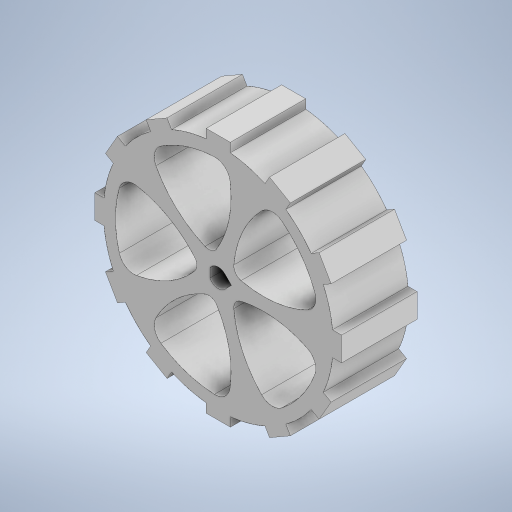
# Autodesk Inventor part: Drive_Wheel
Saved by Autodesk Inventor 2024 (Build 280153000, 153)
## iProperties
Created: 2024-04-15
Part Number: Drive_Wheel
Material: Generic
Document SubType Name: Modeling
Designer: CJ110
Density: 1 g/cm^3
Appearance: Default
Author: CJ110
Autodesk Inventor part; units mm, degrees
ref_plane "YZ Plane" through (0, 0, 0) normal (1, 0, 0) x (0, 1, 0)
ref_plane "XZ Plane" through (0, 0, 0) normal (0, 1, 0) x (-1, 0, 0)
ref_plane "XY Plane" through (0, 0, 0) normal (0, 0, 1) x (1, 0, 0)
sketch "Sketch1" plane through (0, 0, 0) normal (0, 0, 1) x (1, 0, 0)
  circle A0 centre (0, 0) radius 38.1
  circle A1 centre (0, 0) radius 3.1
  line L0 (-2.75, 1.4309) -> (-2.75, -1.4309)
  line L1 (2.192, 2.192) -> (4.3841, 0)
  line L2 (4.3841, 0) -> (2.192, -2.192)
  dimension "d0" = 76.2
  dimension "d1" = 6.2
  dimension "d2" = 2.75
  constraints: 6 end point, 4 point on circle, 2 centre point, 2 coincident, 2 tangent, 1 horizontal alignment, 1 perpendicular, 1 vertical
  measures "d0" diameter of A0
  measures "d1" diameter of A1
  measures "d2" distance from line of L0 point (0, 0)
extrude "Extrusion1" add sketch "Sketch1" along normal blind 25 contours A0 | L0 A1 picked at (-2.8371, 0.2455)
sketch "Sketch3" plane through (0, 0, 25) normal (0, 0, 1) x (1, 0, 0)
  circle A0 centre (0, 0) radius 38.1 projected
  line L0 (4.3841, 0) -> (2.192, -2.192) projected
  arc A1 (-2.75, -1.4309) -> (2.192, -2.192) centre (0, 0) ccw projected
  line L1 (-2.75, -1.4309) -> (-2.75, 1.4309) projected
  arc A2 (2.192, 2.192) -> (-2.75, 1.4309) centre (0, 0) ccw projected
  line L2 (2.192, 2.192) -> (4.3841, 0) projected
  line L3 (0, 0) -> (38.1, 0) construction
  circle A3 centre (0, 0) radius 7.1
  circle A4 centre (0, 0) radius 34.1
  circle A5 centre (0, 0) radius 3.1 construction
  circle A6 centre (27.3278, 10) radius 5
  circle A7 centre (27.3278, -10) radius 5
  line L4 (27.3278, 10) -> (27.3278, 0) construction
  line L5 (27.3278, -10) -> (27.3278, 0) construction
  circle A8 centre (8.2583, 6) radius 3.1078
  circle A9 centre (8.2583, -6) radius 3.1078
  line L6 (8.2583, 6) -> (8.2583, 0) construction
  line L7 (8.2583, -6) -> (8.2583, 0) construction
  arc A10 (7.5566, 2.9724) -> (29.5391, 5.5155) centre (14.9864, 35.0288) ccw
  arc A11 (29.5391, -5.5155) -> (7.5566, -2.9724) centre (14.9864, -35.0288) ccw
  circle A12 centre (17.9553, 22.9001) radius 5
  arc A13 (14.3737, 26.3889) -> (5.1621, 6.2682) centre (37.9454, 3.4284) ccw
  circle A14 centre (-1.0658, 29.0805) radius 5
  circle A15 centre (-16.2308, 24.1531) radius 5
  circle A16 centre (-27.9865, 7.9727) radius 5
  circle A17 centre (-27.9865, -7.9727) radius 5
  circle A18 centre (-16.2308, -24.1531) radius 5
  circle A19 centre (17.9553, -22.9001) radius 5
  circle A20 centre (-1.0658, -29.0805) radius 5
  circle A21 centre (-3.1544, 9.7082) radius 3.1078
  circle A22 centre (-10.2078, 0) radius 3.1078
  circle A23 centre (-3.1544, -9.7082) radius 3.1078
  arc A24 (-0.4919, 8.1053) -> (3.8825, 29.7977) centre (-28.6833, 25.0774) ccw
  arc A25 (5.1621, -6.2682) -> (14.3737, -26.3889) centre (37.9454, -3.4284) ccw
  arc A26 (3.8825, -29.7977) -> (-0.4919, -8.1053) centre (-28.6833, -25.0774) ccw
  arc A27 (-4.3662, -6.8464) -> (-20.6557, -21.8248) centre (8.4652, -37.1477) ccw
  arc A28 (-20.6557, 21.8248) -> (-4.3662, 6.8464) centre (8.4652, 37.1477) ccw
  arc A29 (-7.8606, 2.0369) -> (-27.1396, 12.9005) centre (-32.7137, -19.5301) ccw
  arc A30 (-27.1396, -12.9005) -> (-7.8606, -2.0369) centre (-32.7137, 19.5301) ccw
  line L8 (8.2583, 6) -> (-3.1544, 9.7082) construction
  line L9 (-3.1544, 9.7082) -> (-10.2078, 0) construction
  line L10 (-10.2078, 0) -> (-3.1544, -9.7082) construction
  line L11 (-3.1544, -9.7082) -> (8.2583, -6) construction
  line L12 (17.9553, 22.9001) -> (-1.0658, 29.0805) construction
  line L13 (-16.2308, 24.1531) -> (-27.9865, 7.9727) construction
  line L14 (-27.9865, -7.9727) -> (-16.2308, -24.1531) construction
  line L15 (-1.0658, -29.0805) -> (17.9553, -22.9001) construction
  point P0 (21.0404, -26.8349)
  point P1 (32.0233, -11.7182)
  point P2 (-19.0196, -28.3031)
  point P3 (-1.2489, -34.0771)
  point P4 (-32.7952, 9.3426)
  point P5 (-32.7952, -9.3426)
  point P6 (-1.2489, 34.0771)
  point P7 (-19.0196, 28.3031)
  point P8 (32.0233, 11.7182)
  point P9 (21.0404, 26.8349)
  dimension "d32" = 10
  dimension "d25" = 4
  dimension "d26" = 4
  dimension "d29" = 10
  dimension "d30" = 6
  dimension "d31" = 12
  constraints: 30 point on circle, 26 end point, 18 centre point, 14 equal radius, 14 tangent, 4 equal length, 3 coincident, 2 perpendicular, 2 point on line, 1 collinear, 1 horizontal, 1 horizontal alignment, 1 vertical, 60 other
  measures "d25" radial gap between concentric circles of A5 A3
  measures "d29" distance of L4.start L4.end
  measures "d30" distance of L6.start L6.end
  measures "d31" distance of L10.end L7.start
extrude "Extrusion4" cut sketch "Sketch3" against normal through all contours A8 | A9 | A21 | A13 A12 A4 A6 A10 A8 | A23 | A11 A7 A4 A19 A25 A9 | A22 | A28 A15 A4 A14 A24 A21 | A12 | A6 | A26 A20 A4 A18 A27 A23 | A7 | A19 | A22 A30 A17 A4 A16 A29 | A15 | A14 | A20 | A18 | A16 | A17
sketch "Sketch4" plane through (0, 0, 25) normal (0, 0, 1) x (1, 0, 0)
  arc A0 (-27.1396, 12.9005) -> (-32.7952, 9.3426) centre (-27.9865, 7.9727) ccw projected
  arc A1 (-7.8606, 2.0369) -> (-27.1396, 12.9005) centre (-32.7137, -19.5301) ccw projected
  arc A2 (-7.8606, -2.0369) -> (-7.8606, 2.0369) centre (-10.2078, 0) ccw projected
  arc A3 (-27.1396, -12.9005) -> (-7.8606, -2.0369) centre (-32.7137, 19.5301) ccw projected
  arc A4 (-32.7952, -9.3426) -> (-27.1396, -12.9005) centre (-27.9865, -7.9727) ccw projected
  arc A5 (-32.7952, 9.3426) -> (-32.7952, -9.3426) centre (0, 0) ccw projected
  arc A6 (3.8825, -29.7977) -> (-0.4919, -8.1053) centre (-28.6833, -25.0774) ccw projected
  arc A7 (-1.2489, -34.0771) -> (3.8825, -29.7977) centre (-1.0658, -29.0805) ccw projected
  arc A8 (-19.0196, -28.3031) -> (-1.2489, -34.0771) centre (0, 0) ccw projected
  arc A9 (-20.6557, -21.8248) -> (-19.0196, -28.3031) centre (-16.2308, -24.1531) ccw projected
  arc A10 (-4.3662, -6.8464) -> (-20.6557, -21.8248) centre (8.4652, -37.1477) ccw projected
  arc A11 (-0.4919, -8.1053) -> (-4.3662, -6.8464) centre (-3.1544, -9.7082) ccw projected
  arc A12 (-20.6557, 21.8248) -> (-4.3662, 6.8464) centre (8.4652, 37.1477) ccw projected
  arc A13 (-19.0196, 28.3031) -> (-20.6557, 21.8248) centre (-16.2308, 24.1531) ccw projected
  arc A14 (-1.2489, 34.0771) -> (-19.0196, 28.3031) centre (0, 0) ccw projected
  arc A15 (3.8825, 29.7977) -> (-1.2489, 34.0771) centre (-1.0658, 29.0805) ccw projected
  arc A16 (-0.4919, 8.1053) -> (3.8825, 29.7977) centre (-28.6833, 25.0774) ccw projected
  arc A17 (-4.3662, 6.8464) -> (-0.4919, 8.1053) centre (-3.1544, 9.7082) ccw projected
  arc A18 (29.5391, -5.5155) -> (7.5566, -2.9724) centre (14.9864, -35.0288) ccw projected
  arc A19 (32.0233, -11.7182) -> (29.5391, -5.5155) centre (27.3278, -10) ccw projected
  arc A20 (21.0404, -26.8349) -> (32.0233, -11.7182) centre (0, 0) ccw projected
  arc A21 (14.3737, -26.3889) -> (21.0404, -26.8349) centre (17.9553, -22.9001) ccw projected
  arc A22 (5.1621, -6.2682) -> (14.3737, -26.3889) centre (37.9454, -3.4284) ccw projected
  arc A23 (7.5566, -2.9724) -> (5.1621, -6.2682) centre (8.2583, -6) ccw projected
  arc A24 (7.5566, 2.9724) -> (29.5391, 5.5155) centre (14.9864, 35.0288) ccw projected
  arc A25 (5.1621, 6.2682) -> (7.5566, 2.9724) centre (8.2583, 6) ccw projected
  arc A26 (14.3737, 26.3889) -> (5.1621, 6.2682) centre (37.9454, 3.4284) ccw projected
  arc A27 (21.0404, 26.8349) -> (14.3737, 26.3889) centre (17.9553, 22.9001) ccw projected
  arc A28 (32.0233, 11.7182) -> (21.0404, 26.8349) centre (0, 0) ccw projected
  arc A29 (29.5391, 5.5155) -> (32.0233, 11.7182) centre (27.3278, 10) ccw projected
  circle A30 centre (0, 0) radius 38.1 projected
  line L0 (4.3841, 0) -> (2.192, -2.192) projected
  arc A31 (-2.75, -1.4309) -> (2.192, -2.192) centre (0, 0) ccw projected
  line L1 (-2.75, -1.4309) -> (-2.75, 1.4309) projected
  arc A32 (2.192, 2.192) -> (-2.75, 1.4309) centre (0, 0) ccw projected
  line L2 (2.192, 2.192) -> (4.3841, 0) projected
  line L3 (37.8894, 4) -> (40.8894, 4)
  line L4 (40.8894, 4) -> (40.8894, -4)
  line L5 (40.8894, -4) -> (37.8894, -4)
  line L6 (37.8894, -4) -> (37.8894, 4)
  circle A33 centre (0, 0) radius 38.1 projected
  point P0 (40.8894, 0)
  dimension "d41" = 8
  dimension "d42" = 3
  constraints: 8 end point, 2 parallel, 1 horizontal, 1 horizontal alignment, 1 midpoint, 1 perpendicular, 4 other
  measures "d41" distance between parallel lines of L5 L3
  measures "d42" distance between parallel lines of L6 L4
extrude "Extrusion5" add sketch "Sketch4" against normal up to surface (25 mm away) contours A30 L3 L4 L5
pattern_circular "Circular Pattern2" count 12 over 360 about axis through (0, 0, 0) along (0, 0, 1) of "Extrusion5"
equation "\"d0\" = Wheel_Diameter"
equation "\"d1\" = Axel_Diamter"
equation "\"d2\" = Axel_Cuttout_Dist"
equation "\"d3\" = Wheel_Thickness"
equation "\"Wheel_Diameter\" = 76.2"
equation "\"Axel_Diamter\" = 6.2"
equation "\"Axel_Cuttout_Dist\" = 2.75"
equation "\"Wheel_Thickness\" = 25"
equation "\"Tread_Height\" = 3"
equation "\"Tread_Width\" = 8"
body "Solid1"
